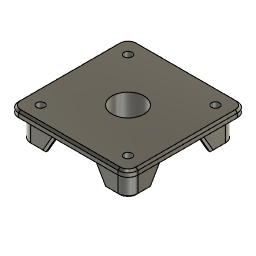
CAM-PoleMount-plug (Autodesk Fusion 360 design; units mm, degrees)
Autodesk Fusion 360 part; units mm, degrees
sketch "Common" plane through (0, 0, 0) normal (0, 0, 1) x (1, 0, 0)
  line L0 (30, -30) -> (-30, -30)
  line L1 (-30, -30) -> (-30, 30)
  line L2 (-30, 30) -> (30, 30)
  line L3 (30, 30) -> (30, -30)
  line L4 (30, -30) -> (-30, 30) construction
  line L5 (-30, -30) -> (30, 30) construction
  circle A0 centre (0, 0) radius 8
  circle A1 centre (0, 0) radius 10
  line L6 (-27, -27) -> (-27, 27)
  line L7 (-27, 27) -> (27, 27)
  line L8 (27, 27) -> (27, -27)
  line L9 (27, -27) -> (-27, -27)
  circle A2 centre (22, -22) radius 2
  circle A3 centre (22, 22) radius 2
  circle A4 centre (-22, 22) radius 2
  circle A5 centre (-22, -22) radius 2
  line L10 (25, -25) -> (-25, -25)
  line L11 (-25, -25) -> (-25, 25)
  line L12 (-25, 25) -> (25, 25)
  line L13 (25, 25) -> (25, -25)
  circle A6 centre (0, 0) radius 24.25
  dimension "d1" = 60
  dimension "d2" = 60
  dimension "d3" = 16
  dimension "d4" = 2
  dimension "d5" = 3
  dimension "d6" = 4
  dimension "d8" = 8
  dimension "d10" = 360
  dimension "d11" = 5
  dimension "d31" = 48.5
  constraint horizontal L0
  constraint perpendicular L0 L1
  constraint parallel L0 L2
  constraint parallel L1 L3
  constraint coincident L4 A0.centre
  constraint coincident L5 A0.centre
  constraint coincident A0.centre A1.centre
  constraint coincident L4 A2.centre
  constraint concentric A0 A6
  measures "d1" distance of L1.end L2.end
  measures "d2" distance of L0.end L1.end
  measures "d3" diameter of A0
  measures "d6" diameter of A2
  measures "d8" distance of L0 A2.centre
  measures "d31" diameter of A6
extrude "Extrude2" add sketch "Common" against normal blind 3 contours L0 L1 L2 L3 in component "Plug"
extrude "Extrude3" add sketch "Common" against normal blind 15 contours L6 L7 L8 L9 in component "Plug"
extrude "Extrude4" add sketch "Common" against normal blind 6 contours L10 L11 L12 L13 | A6 in component "Plug"
sketch "Flange cutout1" plane through (0, 0, 0) normal (0, 1, 0) x (1, 0, 0) in component "Plug"
  line L0 (0, 0) -> (0, 40) construction
  line L1 (0, 6) -> (10, 6)
  line L2 (10, 6) -> (25, 31.9808)
  line L3 (10, 6) -> (37, 6) construction
  line L4 (25, 31.9808) -> (0, 31.9808)
  line L5 (-25, 31.9808) -> (0, 31.9808)
  line L6 (0, 6) -> (-10, 6)
  line L7 (-10, 6) -> (-25, 31.9808)
  dimension "d90" = 40
  dimension "d91" = 10
  dimension "d92" = 6
  dimension "d93" = 30
  dimension "d94" = 60
  constraint coincident L0.start origin
  constraint vertical L0
  constraint horizontal L1
  constraint coincident L0 L1.start
  constraint horizontal L3
  constraint coincident L0 L4.end
  constraint perpendicular L0 L4
  constraint symmetric L0 L1.start L6.start
  constraint symmetric L0 L1.end L6.end
  constraint symmetric L0 L2.end L5.start
  constraint symmetric L0 L4.end L5.end
  measures "d90" distance of L0.start L0.end
  measures "d91" distance of L1.start L1.end
  measures "d92" distance of L0.start L1.start
  measures "d93" distance of L1.end L2.end
  measures "d94" angle of L2 L3
extrude "Extrude6" cut sketch "Flange cutout1" along normal mid plane 100 in component "Plug"
sketch "Flange cutout2" plane through (0, 0, 0) normal (1, 0, 0) x (0, 1, 0) in component "Plug"
  line L0 (-25, -31.9808) -> (0, -31.9808)
  line L1 (0, -6) -> (10, -6)
  line L2 (-10, -6) -> (-25, -31.9808)
  line L3 (0, -6) -> (-10, -6)
  line L4 (-10, -6) -> (-37, -6) construction
  line L5 (0, 0) -> (0, -40) construction
  line L6 (10, -6) -> (25, -31.9808)
  line L7 (25, -31.9808) -> (0, -31.9808)
  point P0 (0.1488, 0.1515)
  dimension "d104" = 40
  dimension "d105" = 10
  dimension "d106" = 6
  dimension "d107" = 30
  dimension "d108" = 60
  constraint coincident L5.start origin
  constraint coincident L1.start L5
  constraint coincident L0.end L5
  constraint perpendicular L0 L5
  measures "d104" distance of L5.start L5.end
  measures "d105" distance of L2.start L1.start
  measures "d106" distance of L5.start L1.start
  measures "d107" distance of L0.start L2.start
  measures "d108" angle of L2 L4
extrude "Extrude7" cut sketch "Flange cutout2" along normal mid plane 200 in component "Plug"
extrude "Extrude5" add sketch "Common" against normal blind 20 contours A1 in component "Plug"
fillet "Fillet1" radius 5 4 edges at (-30, -30, -1.5) (30, -30, -1.5) (30, 30, -1.5) (-30, 30, -1.5) in component "Plug"
fillet "Fillet1" radius 5 4 edges at (-27, 27, -9) (-27, -27, -9) (27, 27, -9) (27, -27, -9) in component "Plug"
fillet "Fillet1" radius 3 4 edges at (-25, 25, -10.5) (25, 25, -10.5) (-25, -25, -10.5) (25, -25, -10.5) in component "Plug"
extrude "Extrude8" cut sketch "Common" against normal blind 3 from surface at -3 contours A6 in component "Plug"
chamfer "Chamfer1" distance 1 angle 45 30 edges at (0, -30, 0) (-28.5355, -28.5355, 0) (-30, 0, 0) (-28.5355, 28.5355, 0) (0, 30, 0) (28.5355, 28.5355, 0) (30, 0, 0) (28.5355, -28.5355, 0) (27, -18.5981, -15) (25.5355, -25.5355, -15) (18.5981, -27, -15) (27, -12.5981, -10.5) (27, 12.5981, -10.5) (25.5355, 25.5355, -15) (27, 18.5981, -15) (18.5981, 27, -15) (-18.5981, 27, -15) (-25.5355, 25.5355, -15) (-27, 18.5981, -15) (-18.5981, -27, -15) (-25.5355, -25.5355, -15) (-27, -18.5981, -15) (-12.5981, -27, -10.5) (-12.5981, 27, -10.5) (12.5981, 27, -10.5) (12.5981, -27, -10.5) (-27, -12.5981, -10.5) (-27, 12.5981, -10.5) (-7.4586, -2.8929, -20) (-22.6089, -8.7692, -6) in component "Plug"
component "Plug" placed x (1, 0, 0) y (0, 1, 0) z (0, 0, 1) at (0, 0, 0)
named bodies: "Plug"
